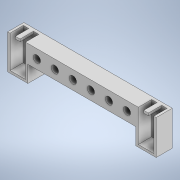
# Autodesk Inventor part: SensorMount
Saved by Autodesk Inventor 2020 (Build 240168000, 168)
## iProperties
Created: 2020-02-20
Part Number: SensorMount
Material: Generic
Document SubType Name: Modeling
Designer: srini
Density: 1 g/cm^3
Appearance: Default
Author: srini
Autodesk Inventor part; units mm, degrees
ref_plane "YZ Plane" through (0, 0, 0) normal (1, 0, 0) x (0, 1, 0)
ref_plane "XZ Plane" through (0, 0, 0) normal (0, 1, 0) x (-1, 0, 0)
ref_plane "XY Plane" through (0, 0, 0) normal (0, 0, 1) x (1, 0, 0)
sketch "Sketch1" plane through (0, 0, 0) normal (0, 0, 1) x (1, 0, 0)
  line L0 (-52.362, 12.7) -> (-38.1, 12.7)
  line L1 (-38.1, 12.7) -> (-38.1, -11.722)
  line L2 (-38.1, -11.722) -> (-52.362, -11.722)
  line L3 (-52.362, -11.722) -> (-52.362, 12.7)
  line L4 (-38.1, 12.7) -> (38.1, 12.7)
  line L5 (38.1, 12.7) -> (38.1, 0)
  line L6 (38.1, 0) -> (-38.1, 0)
  line L7 (-38.1, 0) -> (-38.1, 12.7)
  line L8 (38.1, 12.7) -> (52.362, 12.7)
  line L9 (52.362, 12.7) -> (52.362, -11.722)
  line L10 (52.362, -11.722) -> (38.1, -11.722)
  line L11 (38.1, -11.722) -> (38.1, 12.7)
  point P0 (0, 0)
  dimension "d0" = 14.262
  dimension "d1" = 12.7
  dimension "d2" = 24.422
  dimension "d3" = 76.2
  dimension "d4" = 38.1
  constraints: 24 end point, 6 parallel, 3 horizontal, 3 perpendicular, 2 collinear, 1 midpoint
  measures "d0" distance between parallel lines of L1 L3
  measures "d1" distance between parallel lines of L6 L4
  measures "d2" distance between parallel lines of L2 L0
  measures "d3" distance between parallel lines of L5 L1
  measures "d4" distance from line of point (0, 0) L1
extrude "Extrusion1" add sketch "Sketch1" along normal blind 11.398
sketch "Sketch2" plane through (0, 0, 11.398) normal (0, 0, 1) x (1, 0, 0)
  line L0 (-50.692, 11.03) -> (-39.77, 11.03)
  line L1 (-39.77, 11.03) -> (-39.77, -10.052)
  line L2 (-39.77, -10.052) -> (-50.692, -10.052)
  line L3 (-50.692, -10.052) -> (-50.692, 11.03)
  line L4 (39.77, 11.03) -> (50.692, 11.03)
  line L5 (50.692, 11.03) -> (50.692, -10.052)
  line L6 (50.692, -10.052) -> (39.77, -10.052)
  line L7 (39.77, -10.052) -> (39.77, 11.03)
  line L8 (52.362, 12.7) -> (-52.362, 12.7) projected
  line L9 (-52.362, 12.7) -> (-52.362, -11.722) projected
  line L10 (52.362, -11.722) -> (52.362, 12.7) projected
  line L11 (-50.692, 18.6326) -> (-46.882, 18.6326)
  line L12 (-46.882, 18.6326) -> (-46.882, 11.03)
  line L13 (-46.882, 11.03) -> (-50.692, 11.03)
  line L14 (-50.692, 11.03) -> (-50.692, 18.6326)
  line L15 (-43.58, 18.6326) -> (-39.77, 18.6326)
  line L16 (-39.77, 18.6326) -> (-39.77, 11.03)
  line L17 (-39.77, 11.03) -> (-43.58, 11.03)
  line L18 (-43.58, 11.03) -> (-43.58, 18.6326)
  line L19 (39.77, 18.4615) -> (43.58, 18.4615)
  line L20 (43.58, 18.4615) -> (43.58, 11.03)
  line L21 (43.58, 11.03) -> (39.77, 11.03)
  line L22 (39.77, 11.03) -> (39.77, 18.4615)
  line L23 (46.882, 18.4615) -> (50.692, 18.4615)
  line L24 (50.692, 18.4615) -> (50.692, 11.03)
  line L25 (50.692, 11.03) -> (46.882, 11.03)
  line L26 (46.882, 11.03) -> (46.882, 18.4615)
  point P0 (0, 0)
  point P1 (-43.58, 12.7)
  point P2 (-46.882, 12.7)
  point P3 (46.882, 12.7)
  point P4 (43.58, 12.7)
  dimension "d7" = 10.922
  dimension "d8" = 21.082
  dimension "d9" = 1.67
  dimension "d10" = 1.67
  dimension "d11" = 1.67
  dimension "d12" = 3.302
  constraints: 48 end point, 12 parallel, 8 collinear, 6 horizontal, 6 perpendicular, 4 equal length, 4 point on line
  measures "d7" distance of L0.start L0.end
  measures "d8" distance of L2.end L0.start
  measures "d9" distance between parallel lines of L0 L8
  measures "d10" distance between parallel lines of L9 L3
  measures "d11" distance between parallel lines of L5 L10
  measures "d12" distance between parallel lines of L18 L12
extrude "Extrusion2" cut sketch "Sketch2" against normal blind 9.398 contours L14 L8 L12 L0 | L0 L1 L2 L3 | L22 L19 L20 L8 | L8 L20 L4 L22 | L14 L11 L12 L8 | L18 L8 L16 L0 | L18 L15 L16 L8 | L4 L5 L6 L7 | L26 L23 L24 L8 | L8 L24 L4 L26
sketch "Sketch3" plane through (0, 0, 11.398) normal (0, 0, 1) x (1, 0, 0)
  circle A0 centre (-31.75, 6.35) radius 2.5781
  line L0 (-38.1, 0) -> (38.1, 0) projected
  circle A1 centre (-19.05, 6.35) radius 2.5781
  circle A2 centre (-6.35, 6.35) radius 2.5781
  circle A3 centre (6.35, 6.35) radius 2.5781
  circle A4 centre (19.05, 6.35) radius 2.5781
  circle A5 centre (31.75, 6.35) radius 2.5781
  point P0 (0, 0)
  dimension "d15" = 5.1562
  dimension "d16" = 6.35
  dimension "d17" = 31.75
  dimension "d23" = 12.7
  constraints: 6 centre point, 1 horizontal, 10 other
  measures "d15" diameter of A0
  measures "d16" distance from line of A0.centre L0
  measures "d17" horizontal distance of A0.centre point (0, 0)
  measures "d23" distance of A0.centre A1.centre
extrude "Extrusion3" cut sketch "Sketch3" against normal through all
sketch "Sketch5" plane through (0, 0, 0) normal (0, 0, -1) x (-1, 0, 0)
  circle A0 centre (31.75, 6.35) radius 2.5781 projected
  line L0 (28.8849, 11.3125) -> (34.6151, 11.3125)
  line L1 (34.6151, 11.3125) -> (37.4802, 6.35)
  line L2 (37.4802, 6.35) -> (34.6151, 1.3875)
  line L3 (34.6151, 1.3875) -> (28.8849, 1.3875)
  line L4 (28.8849, 1.3875) -> (26.0198, 6.35)
  line L5 (26.0198, 6.35) -> (28.8849, 11.3125)
  line L6 (-52.362, 12.7) -> (52.362, 12.7) projected
  line L7 (16.1849, 11.3125) -> (21.9151, 11.3125)
  line L8 (21.9151, 11.3125) -> (24.7802, 6.35)
  line L9 (24.7802, 6.35) -> (21.9151, 1.3875)
  line L10 (21.9151, 1.3875) -> (16.1849, 1.3875)
  line L11 (16.1849, 1.3875) -> (13.3198, 6.35)
  line L12 (13.3198, 6.35) -> (16.1849, 11.3125)
  line L13 (3.4849, 11.3125) -> (9.2151, 11.3125)
  line L14 (9.2151, 11.3125) -> (12.0802, 6.35)
  line L15 (12.0802, 6.35) -> (9.2151, 1.3875)
  line L16 (9.2151, 1.3875) -> (3.4849, 1.3875)
  line L17 (3.4849, 1.3875) -> (0.6198, 6.35)
  line L18 (0.6198, 6.35) -> (3.4849, 11.3125)
  line L19 (-9.2151, 11.3125) -> (-3.4849, 11.3125)
  line L20 (-3.4849, 11.3125) -> (-0.6198, 6.35)
  line L21 (-0.6198, 6.35) -> (-3.4849, 1.3875)
  line L22 (-3.4849, 1.3875) -> (-9.2151, 1.3875)
  line L23 (-9.2151, 1.3875) -> (-12.0802, 6.35)
  line L24 (-12.0802, 6.35) -> (-9.2151, 11.3125)
  line L25 (-21.9151, 11.3125) -> (-16.1849, 11.3125)
  line L26 (-16.1849, 11.3125) -> (-13.3198, 6.35)
  line L27 (-13.3198, 6.35) -> (-16.1849, 1.3875)
  line L28 (-16.1849, 1.3875) -> (-21.9151, 1.3875)
  line L29 (-21.9151, 1.3875) -> (-24.7802, 6.35)
  line L30 (-24.7802, 6.35) -> (-21.9151, 11.3125)
  line L31 (-34.6151, 11.3125) -> (-28.8849, 11.3125)
  line L32 (-28.8849, 11.3125) -> (-26.0198, 6.35)
  line L33 (-26.0198, 6.35) -> (-28.8849, 1.3875)
  line L34 (-28.8849, 1.3875) -> (-34.6151, 1.3875)
  line L35 (-34.6151, 1.3875) -> (-37.4802, 6.35)
  line L36 (-37.4802, 6.35) -> (-34.6151, 11.3125)
  point P0 (19.05, 6.35)
  point P1 (6.35, 6.35)
  point P2 (-6.35, 6.35)
  point P3 (-19.05, 6.35)
  point P4 (-31.75, 6.35)
  dimension "d28" = 9.925
  dimension "d31" = 12.7
  constraints: 72 end point, 2 horizontal, 1 coincident, 78 other
  measures "d28" distance between parallel lines of L3 L0
  measures "d31" distance of point (31.75, 6.35) point (19.05, 6.35)
extrude "Extrusion4" cut sketch "Sketch5" against normal blind 3.175 contours A0 | L0 L1 L2 L3 L4 L5 | L7 L8 L9 L10 L11 L12 | L13 L14 L15 L16 L17 L18 | L19 L20 L21 L22 L23 L24 | L25 L26 L27 L28 L29 L30 | L31 L32 L33 L34 L35 L36
sketch "Sketch6" plane through (0, 0, 3.175) normal (0, 0, -1) x (-1, 0, 0)
  line L0 (-34.3281, 11.3125) -> (-29.1719, 11.3125)
  line L1 (-29.1719, 11.3125) -> (-29.1719, 1.3875)
  line L2 (-29.1719, 1.3875) -> (-34.3281, 1.3875)
  line L3 (-34.3281, 1.3875) -> (-34.3281, 11.3125)
  circle A0 centre (-31.75, 6.35) radius 2.5781 construction
  line L4 (-34.3281, 11.3125) -> (-29.1719, 1.3875) construction
  line L5 (-29.1719, 11.3125) -> (-34.3281, 1.3875) construction
  line L6 (-34.6151, 11.3125) -> (-28.8849, 11.3125) projected
  line L7 (-52.362, 12.7) -> (52.362, 12.7) projected
  line L8 (-21.6281, 11.3125) -> (-16.4719, 11.3125)
  line L9 (-16.4719, 11.3125) -> (-16.4719, 1.3875)
  line L10 (-16.4719, 1.3875) -> (-21.6281, 1.3875)
  line L11 (-21.6281, 1.3875) -> (-21.6281, 11.3125)
  line L12 (-21.6281, 11.3125) -> (-16.4719, 1.3875) construction
  line L13 (-16.4719, 11.3125) -> (-21.6281, 1.3875) construction
  line L14 (-8.9281, 11.3125) -> (-3.7719, 11.3125)
  line L15 (-3.7719, 11.3125) -> (-3.7719, 1.3875)
  line L16 (-3.7719, 1.3875) -> (-8.9281, 1.3875)
  line L17 (-8.9281, 1.3875) -> (-8.9281, 11.3125)
  line L18 (-8.9281, 11.3125) -> (-3.7719, 1.3875) construction
  line L19 (-3.7719, 11.3125) -> (-8.9281, 1.3875) construction
  line L20 (3.7719, 11.3125) -> (8.9281, 11.3125)
  line L21 (8.9281, 11.3125) -> (8.9281, 1.3875)
  line L22 (8.9281, 1.3875) -> (3.7719, 1.3875)
  line L23 (3.7719, 1.3875) -> (3.7719, 11.3125)
  line L24 (3.7719, 11.3125) -> (8.9281, 1.3875) construction
  line L25 (8.9281, 11.3125) -> (3.7719, 1.3875) construction
  line L26 (16.4719, 11.3125) -> (21.6281, 11.3125)
  line L27 (21.6281, 11.3125) -> (21.6281, 1.3875)
  line L28 (21.6281, 1.3875) -> (16.4719, 1.3875)
  line L29 (16.4719, 1.3875) -> (16.4719, 11.3125)
  line L30 (16.4719, 11.3125) -> (21.6281, 1.3875) construction
  line L31 (21.6281, 11.3125) -> (16.4719, 1.3875) construction
  line L32 (29.1719, 11.3125) -> (34.3281, 11.3125)
  line L33 (34.3281, 11.3125) -> (34.3281, 1.3875)
  line L34 (34.3281, 1.3875) -> (29.1719, 1.3875)
  line L35 (29.1719, 1.3875) -> (29.1719, 11.3125)
  line L36 (29.1719, 11.3125) -> (34.3281, 1.3875) construction
  line L37 (34.3281, 11.3125) -> (29.1719, 1.3875) construction
  point P0 (0, 0)
  point P1 (-19.05, 6.35)
  point P2 (-6.35, 6.35)
  point P3 (6.35, 6.35)
  point P4 (19.05, 6.35)
  point P5 (31.75, 6.35)
  dimension "d40" = 12.7
  constraints: 72 end point, 12 midpoint, 2 horizontal, 2 parallel, 1 collinear, 1 perpendicular, 1 tangent, 55 other
  measures "d40" distance of L0.start L8.start
extrude "Extrusion5" cut sketch "Sketch6" against normal blind 0.2
sketch "Sketch7" plane through (0, 0, 3.375) normal (0, 0, -1) x (-1, 0, 0)
  line L0 (-29.1719, 3.7719) -> (-34.3281, 3.7719)
  line L1 (-34.3281, 3.7719) -> (-34.3281, 8.9281)
  line L2 (-34.3281, 8.9281) -> (-29.1719, 8.9281)
  line L3 (-29.1719, 8.9281) -> (-29.1719, 3.7719)
  circle A0 centre (-31.75, 6.35) radius 2.5781 construction
  line L4 (-29.1719, 3.7719) -> (-34.3281, 8.9281) construction
  line L5 (-34.3281, 3.7719) -> (-29.1719, 8.9281) construction
  line L6 (-52.362, 12.7) -> (52.362, 12.7) projected
  line L7 (-16.4719, 3.7719) -> (-21.6281, 3.7719)
  line L8 (-21.6281, 3.7719) -> (-21.6281, 8.9281)
  line L9 (-21.6281, 8.9281) -> (-16.4719, 8.9281)
  line L10 (-16.4719, 8.9281) -> (-16.4719, 3.7719)
  line L11 (-16.4719, 3.7719) -> (-21.6281, 8.9281) construction
  line L12 (-21.6281, 3.7719) -> (-16.4719, 8.9281) construction
  line L13 (-3.7719, 3.7719) -> (-8.9281, 3.7719)
  line L14 (-8.9281, 3.7719) -> (-8.9281, 8.9281)
  line L15 (-8.9281, 8.9281) -> (-3.7719, 8.9281)
  line L16 (-3.7719, 8.9281) -> (-3.7719, 3.7719)
  line L17 (-3.7719, 3.7719) -> (-8.9281, 8.9281) construction
  line L18 (-8.9281, 3.7719) -> (-3.7719, 8.9281) construction
  line L19 (8.9281, 3.7719) -> (3.7719, 3.7719)
  line L20 (3.7719, 3.7719) -> (3.7719, 8.9281)
  line L21 (3.7719, 8.9281) -> (8.9281, 8.9281)
  line L22 (8.9281, 8.9281) -> (8.9281, 3.7719)
  line L23 (8.9281, 3.7719) -> (3.7719, 8.9281) construction
  line L24 (3.7719, 3.7719) -> (8.9281, 8.9281) construction
  line L25 (21.6281, 3.7719) -> (16.4719, 3.7719)
  line L26 (16.4719, 3.7719) -> (16.4719, 8.9281)
  line L27 (16.4719, 8.9281) -> (21.6281, 8.9281)
  line L28 (21.6281, 8.9281) -> (21.6281, 3.7719)
  line L29 (21.6281, 3.7719) -> (16.4719, 8.9281) construction
  line L30 (16.4719, 3.7719) -> (21.6281, 8.9281) construction
  line L31 (34.3281, 3.7719) -> (29.1719, 3.7719)
  line L32 (29.1719, 3.7719) -> (29.1719, 8.9281)
  line L33 (29.1719, 8.9281) -> (34.3281, 8.9281)
  line L34 (34.3281, 8.9281) -> (34.3281, 3.7719)
  line L35 (34.3281, 3.7719) -> (29.1719, 8.9281) construction
  line L36 (29.1719, 3.7719) -> (34.3281, 8.9281) construction
  point P0 (0, 0)
  point P1 (-19.05, 6.35)
  point P2 (-6.35, 6.35)
  point P3 (6.35, 6.35)
  point P4 (19.05, 6.35)
  point P5 (31.75, 6.35)
  dimension "d49" = 12.7
  constraints: 72 end point, 12 midpoint, 2 horizontal, 2 parallel, 2 tangent, 1 perpendicular, 55 other
  measures "d49" distance of L0.start L7.start
extrude "Extrusion6" cut sketch "Sketch7" against normal blind 0.2
equation "\"d0\" = SensorWide + 2 * WallThick"
equation "\"d2\" = SensorTall + 2 * WallThick"
equation "\"d4\" = 0.5 * d3"
equation "\"d7\" = SensorWide"
equation "\"d8\" = SensorTall"
equation "\"d9\" = WallThick"
equation "\"d10\" = WallThick"
equation "\"d11\" = WallThick"
equation "\"d12\" = SensorCableTabWide"
equation "\"d13\" = SensorThick"
equation "\"WallThick\" = 1.67"
equation "\"SensorWide\" = 10.922"
equation "\"SensorTall\" = 21.082"
equation "\"SensorThick\" = 9.398"
equation "\"SensorCableTabWide\" = 3.302"
body "Solid1"
